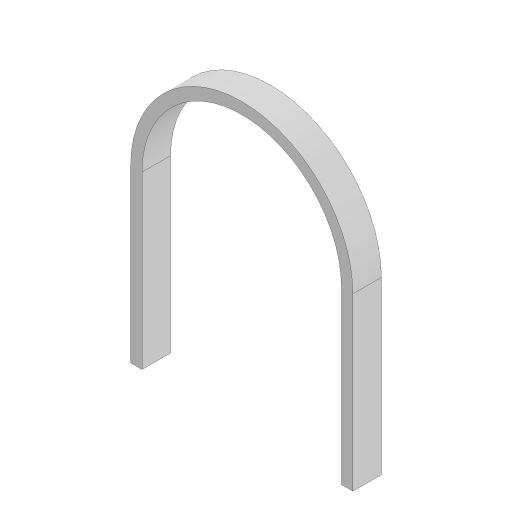
# Autodesk Inventor part: Team29_TubeHolder
Saved by Autodesk Inventor 2023 (Build 270158000, 158)
## iProperties
Created: 2023-02-17
Part Number: Team29_TubeHolder
Material: Generic
Document SubType Name: Modeling
Designer: Fariha
Density: 1 g/cm^3
Appearance: Default
Author: Fariha
Autodesk Inventor part; units mm, degrees
ref_plane "YZ Plane" through (0, 0, 0) normal (1, 0, 0) x (0, 1, 0)
ref_plane "XZ Plane" through (0, 0, 0) normal (0, 1, 0) x (-1, 0, 0)
ref_plane "XY Plane" through (0, 0, 0) normal (0, 0, 1) x (1, 0, 0)
sketch "Sketch1" plane through (0, 0, 0) normal (0, 0, 1) x (1, 0, 0)
  arc A0 (17.5, 0) -> (-17.5, 0) centre (0, 0) ccw
  arc A1 (19.5, 0) -> (-19.5, 0) centre (0, 0) ccw
  line L0 (-19.5, 0) -> (-17.5, 0)
  line L1 (-17.5, 0) -> (-17.5, -10)
  line L2 (-17.5, -10) -> (-19.5, -10)
  line L3 (-19.5, -10) -> (-19.5, 0)
  line L4 (17.5, 0) -> (19.5, 0)
  line L5 (19.5, 0) -> (19.5, -10)
  line L6 (19.5, -10) -> (17.5, -10)
  line L7 (17.5, -10) -> (17.5, 0)
  dimension "d0" = 17.5
  dimension "d1" = 19.5
  dimension "d2" = 10
  dimension "d3" = 10
  dimension "d4" = 2
  dimension "d5" = 2
  dimension "d6" = 19.5
  dimension "d7" = 19.5
  constraints: 16 end point, 4 parallel, 4 point on circle, 2 centre point, 2 coincident, 2 horizontal, 2 perpendicular
  measures "d0" distance of L4.start point (0, 0)
  measures "d1" distance of A1.start point (0, 0)
  measures "d2" distance of L0.end L1.end
  measures "d3" distance of L4.end L5.end
  measures "d4" distance between parallel lines of L3 L1
  measures "d5" distance between parallel lines of L5 L7
  measures "d6" distance from line of L3 point (0, 0)
  measures "d7" distance from line of L5 point (0, 0)
extrude "Extrusion1" add sketch "Sketch1" along normal blind 5
sketch "Sketch2" plane through (17.5, -10, 0) normal (0, -1, 0) x (1, 0, 0)
  line L0 (-35, 0) -> (-35, 5) projected
  line L1 (-37, 5) -> (-35, 5)
  line L2 (-35, 5) -> (-35, 0)
  line L3 (-35, 0) -> (-37, 0)
  line L4 (-37, 0) -> (-37, 5)
  line L5 (2, 0) -> (0, 0)
  line L6 (0, 0) -> (0, 5)
  line L7 (0, 5) -> (2, 5)
  line L8 (2, 5) -> (2, 0)
  point P0 (-17.5, 0)
  dimension "d10" = 2
  dimension "d11" = 5
  dimension "d12" = 2
  dimension "d13" = 5
  constraints: 16 end point, 4 parallel, 2 horizontal, 2 perpendicular
  measures "d10" distance of L0.start L3.end
  measures "d11" distance of L1.end L0.start
  measures "d12" distance of L6.end L7.end
  measures "d13" distance of L5.end L6.end
extrude "Extrusion2" add sketch "Sketch2" along normal blind 20
body "Solid1"
